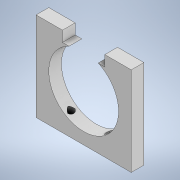
# Autodesk Inventor part: Motor_Mount_Backplate
Saved by Autodesk Inventor 2022 (Build 260153000, 153)
## iProperties
Created: 2022-01-23
Part Number: Motor_Mount_Backplate
Material: Generic
Document SubType Name: Modeling
Designer: Mlees
Density: 1 g/cm^3
Appearance: Default
Author: Mlees
Autodesk Inventor part; units mm, degrees
ref_plane "YZ Plane" through (0, 0, 0) normal (1, 0, 0) x (0, 1, 0)
ref_plane "XZ Plane" through (0, 0, 0) normal (0, 1, 0) x (-1, 0, 0)
ref_plane "XY Plane" through (0, 0, 0) normal (0, 0, 1) x (1, 0, 0)
sketch "Sketch1" plane through (0, 0, 0) normal (0, 1, 0) x (-1, 0, 0)
  line L0 (0, 0) -> (45, 0)
  line L1 (45, 0) -> (45, -6)
  line L2 (45, -6) -> (0, -6)
  line L3 (0, -6) -> (0, 0)
  dimension "d0" = 45
  dimension "d1" = 6
  constraints: 8 end point, 2 parallel, 1 horizontal, 1 perpendicular
  measures "d0" distance of L1.end L2.end
  measures "d1" distance of L0.end L1.end
extrude "Extrusion1" add sketch "Sketch1" along normal blind 42
sketch "Sketch2" plane through (-45, 0, 0) normal (0, 0, 1) x (1, 0, 0)
  line L0 (45, 42) -> (0, 42) projected
  line L1 (22.5, 42) -> (12.5, 42)
  line L2 (22.5, 42) -> (32.5, 42)
  line L3 (32.5, 42) -> (32.5, 37)
  line L4 (32.5, 37) -> (12.5, 37)
  line L5 (12.5, 37) -> (12.5, 42)
  point P0 (45, 0)
  dimension "d4" = 10
  dimension "d5" = 10
  dimension "d6" = 5
  constraints: 10 end point, 3 perpendicular, 2 point on line, 1 midpoint
  measures "d4" distance of L1.start L1.end
  measures "d5" distance of L1.start L2.end
  measures "d6" distance of L2.end L3.end
extrude "Extrusion2" cut sketch "Sketch2" against normal up to surface (6 mm away)
sketch "Sketch3" plane through (0, 0, 0) normal (0, -1, 0) x (1, 0, 0)
  line L0 (-12.5, 0) -> (-32.5, 0) projected
  line L1 (-22.5, 0) -> (-22.5, -3)
  line L2 (-22.5, -3) -> (-12.5, -3)
  line L3 (-22.5, -3) -> (-32.5, -3)
  point P0 (0, 0)
  dimension "d9" = 3
  dimension "d10" = 10
  dimension "d11" = 10
  constraints: 6 end point, 2 coincident, 1 horizontal, 1 midpoint, 1 perpendicular, 1 vertical
  measures "d9" distance of L1.start L1.end
  measures "d10" distance of L1.end L2.end
  measures "d11" distance of L1.end L3.end
hole "Hole1" at (-12.5, 0, -3) at (-32.5, 0, -3) direction (0, 1, 0) diameter 4.5 depth 8 tip angle 118
sketch "Sketch4" plane through (-45, 0, 0) normal (0, 0, 1) x (1, 0, 0)
  line L0 (45, 0) -> (0, 0) projected
  line L1 (22.5, 0) -> (22.5, 22)
  circle A0 centre (22.5, 22) radius 16.5
  dimension "d19" = 22
  dimension "d20" = 33
  constraints: 2 end point, 1 centre point, 1 coincident, 1 midpoint, 1 vertical
  measures "d19" distance of L1.start L1.end
  measures "d20" diameter of A0
extrude "Extrusion3" cut sketch "Sketch4" against normal through all
body "Solid1"
